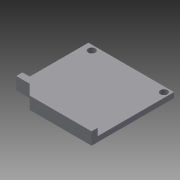
# Autodesk Inventor part: XCarriageFanMount
Saved by Autodesk Inventor 2015 (Build 190159000, 159)
## iProperties
Created: 2014-12-07
Part Number: XCarriageFanMount
Material: Generic
Document SubType Name: Modeling
Designer: Jack
Density: 1 g/cm^3
Appearance: Default
Author: Jack
Autodesk Inventor part; units mm, degrees
ref_plane "YZ Plane" through (0, 0, 0) normal (1, 0, 0) x (0, 1, 0)
ref_plane "XZ Plane" through (0, 0, 0) normal (0, 1, 0) x (-1, 0, 0)
ref_plane "XY Plane" through (0, 0, 0) normal (0, 0, 1) x (1, 0, 0)
sketch "Sketch4" plane through (0, 0, 0) normal (0, 0, 1) x (1, 0, 0)
  line L0 (0, 0) -> (30, 0)
  line L1 (0, 0) -> (-5, 5)
  line L2 (-5, 5) -> (-11.5, 5)
  line L3 (30, 0) -> (30, 40)
  line L4 (30, 40) -> (-11.5, 40)
  line L5 (-11.5, 40) -> (-11.5, 5)
  dimension "d16" = 30
  dimension "d17" = 5
  dimension "d18" = 135
  dimension "d19" = 6.5
  dimension "d20" = 40
  constraints: 12 end point, 2 horizontal, 2 perpendicular, 1 vertical
  measures "d16" distance of L0.start L0.end
  measures "d17" horizontal distance of L0.start L1.end
  measures "d18" angle of L0 L1
  measures "d19" distance of L1.end L2.end
  measures "d20" distance of L0.end L3.end
extrude "Extrusion4" add sketch "Sketch4" along normal blind 2.5
sketch "Sketch5" plane through (0, 0, 2.5) normal (0, 0, 1) x (1, 0, 0)
  line L0 (0, 0) -> (30, 0) projected
  line L1 (30, 0) -> (30, 40) projected
  line L2 (-11.5, 40) -> (-11.5, 5) projected
  line L3 (-11.5, 5) -> (-5, 5) projected
  line L4 (-5, 5) -> (0, 0) projected
  line L5 (-11.5, 8) -> (-3.7574, 8)
  line L6 (-3.7574, 8) -> (1.2426, 3)
  line L7 (1.2426, 3) -> (30, 3)
  dimension "d23" = 3
  dimension "d24" = 3
  dimension "d25" = 3
  constraints: 6 end point, 2 parallel, 2 point on line, 1 horizontal
  measures "d23" distance between parallel lines of L6 L4
  measures "d24" distance between parallel lines of L0 L7
  measures "d25" distance between parallel lines of L5 L3
extrude "Extrusion5" add sketch "Sketch5" along normal blind 3.5
sketch "Sketch6" plane through (0, 0, 2.5) normal (0, 0, 1) x (1, 0, 0)
  line L0 (-11.5, 8) -> (-3.7574, 8) projected
  line L1 (1.2426, 3) -> (30, 3) projected
  line L2 (30, 3) -> (30, 40) projected
  line L3 (-11.5, 40) -> (-11.5, 8) projected
  circle A0 centre (-7.4, 37.5) radius 1.75
  circle A1 centre (27.6, 37.5) radius 1.75
  point P0 (0, 0)
  dimension "d28" = 29.5
  dimension "d29" = 4.1
  dimension "d30" = 3.5
  dimension "d31" = 3.5
  dimension "d32" = 2.4
  dimension "d33" = 34.5
  dimension "d36" = 6
  dimension "d37" = 6
  constraints: 2 centre point
  measures "d28" distance from line of L0 A0.centre
  measures "d29" distance from line of L3 A0.centre
  measures "d30" diameter of A0
  measures "d31" diameter of A1
  measures "d32" distance from line of L2 A1.centre
  measures "d33" distance from line of L1 A1.centre
extrude "Extrusion6" cut sketch "Sketch6" against normal up to next
body "Solid2"
